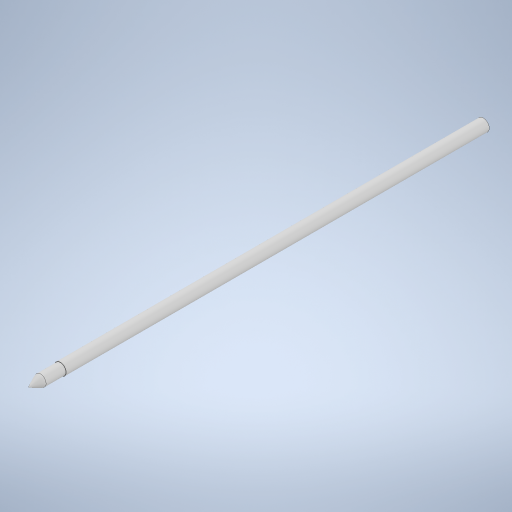
# Autodesk Inventor part: 筆芯
Saved by Autodesk Inventor 2024.2 (Build 282272000, 272)
## iProperties
Created: 2024-04-18
Part Number: 筆芯
Material: 一般
Document SubType Name: Modeling
Designer: User
Density: 1 g/cm^3
Appearance: 預設
Author: User
Autodesk Inventor part; units mm, degrees
ref_plane "YZ Plane" through (0, 0, 0) normal (1, 0, 0) x (0, 1, 0)
ref_plane "XZ Plane" through (0, 0, 0) normal (0, 1, 0) x (-1, 0, 0)
ref_plane "XY Plane" through (0, 0, 0) normal (0, 0, 1) x (1, 0, 0)
sketch "草圖1" plane through (0, 0, 0) normal (0, 1, 0) x (-1, 0, 0)
  line L0 (0, 0) -> (0, -115)
  line L1 (0, -115) -> (1.5, -115)
  line L2 (1.5, -115) -> (1.5, -8)
  line L3 (1.5, -8) -> (1.5, -8.1)
  line L4 (1.5, -8) -> (1.4, -8)
  line L5 (1.4, -8) -> (1.4, -3)
  line L6 (0, 0) -> (0.0831, 0) construction
  line L7 (0.0831, 0) -> (0.4369, -0.6984) construction
  line L8 (0.4369, -0.6984) -> (0.929, -1.7279) construction
  line L9 (0.929, -1.7279) -> (1.4, -2.7133) construction
  line L10 (1.4, -2.7133) -> (1.4, -3) construction
  spline S0 degree 4 poles (0, 0) (0.0831, 0) (0.4369, -0.6984) (0.929, -1.7279) (1.4, -2.7133) (1.4, -3) knots 0 0 0 0 0 1 2 2 2 2 2
  line L11 (1.5, -8) -> (1.5, -21)
  arc A0 (1.5836, -22.9983) -> (1.5, -21) centre (1.5558, -21.9985) ccw
  dimension "d0" = 115
  dimension "d1" = 1.5
  dimension "d2" = 107
  dimension "d4" = 0.1
  dimension "d5" = 5
  dimension "d8" = 13
  dimension "d9" = 2
  dimension "d10" = 1.0001
  constraints: 14 end point, 2 point on circle, 2 point on line, 2 vertical, 1 centre point, 1 horizontal, 1 parallel, 1 perpendicular, 3 other
  measures "d0" distance of L0.start L0.end
  measures "d1" distance of L0.end L1.end
  measures "d2" distance of L1.end L2.end
  measures "d4" distance of L2.end L4.end
  measures "d5" distance of L4.end L5.end
  measures "d8" distance of L2.end L11.end
  measures "d9" distance of L11.end A0.start
  measures "d10" radius of A0
revolve "迴轉1" add sketch "草圖1" angle 360 about axis through (0, 0, 0) along (0, 0, -1)
sketch "草圖2" plane through (0, 0, -115) normal (0, 0, -1) x (-1, 0, 0)
  point P0 (0, 0)
  point P1 (0, 0)
  constraints: 1 coincident
hole "孔1" at (0, 0, -115) direction (0, 0, 1) diameter 2.5 depth 105 tip angle 118
